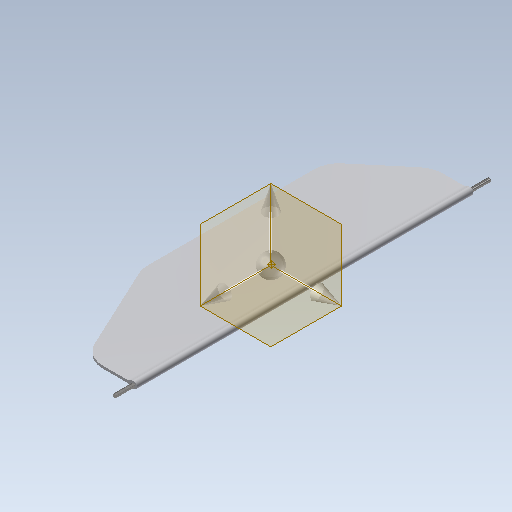
# Autodesk Inventor part: tail2
Saved by Autodesk Inventor 2020 (Build 240168000, 168)
## iProperties
Created: 2016-11-20
Part Number: tail2
Material: Generic
Document SubType Name: Modeling
Designer: jous
Density: 1 g/cm^3
Appearance: Default
Mass: 312.78 g
Surface Area: 1473.46 cm^2
Volume: 312.78 cm^3
sail_heightx: 1000.000 mm
tail_offsetx: 100.000 mm
Author: jous
Autodesk Inventor part; units mm, degrees
ref_plane "YZ Plane" through (0, 0, 0) normal (1, 0, 0) x (0, 1, 0)
ref_plane "XZ Plane" through (0, 0, 0) normal (0, 1, 0) x (-1, 0, 0)
ref_plane "XY Plane" through (0, 0, 0) normal (0, 0, 1) x (1, 0, 0)
sketch "Sketch1" plane through (0, 0, 0) normal (0, 0, 1) x (1, 0, 0)
  circle A0 centre (0, 0) radius 5.5
  circle A1 centre (0, 0) radius 3
  dimension "d0" = 11
  dimension "d1" = 6
  constraints: 2 centre point, 2 coincident
  measures "d0" diameter of A0
  measures "d1" diameter of A1
extrude "tube" add sketch "Sketch1" along normal blind 530
sketch "Sketch2" plane through (0, 0, 0) normal (0, 1, 0) x (-1, 0, 0)
  line L0 (0, 0) -> (150, 0)
  line L1 (150, 0) -> (150, 530)
  line L2 (150, 530) -> (0, 530)
  line L3 (0, 530) -> (0, 0)
  line L4 (75, 0) -> (165.4178, 0) construction
  line L5 (74, 530) -> (150, 367.0175)
  line L6 (74, 530) -> (253.8313, 530) construction
  line L7 (150, 77.1972) -> (58, 0)
  point P0 (150, 333)
  dimension "d4" = 150
  dimension "d5" = 530
  dimension "d9" = 65
  dimension "d16" = 74
  dimension "d17" = 58
  dimension "d18" = 40
  constraints: 16 end point, 5 point on line, 3 horizontal, 2 midpoint, 2 parallel, 1 equal length, 1 perpendicular
  measures "d4" distance of L2.end L1.end
  measures "d5" distance of L0.end L1.end
  measures "d9" angle of L5 L6
  measures "d16" distance of L2.end L5.start
  measures "d17" distance from line of L3 L7.end
  measures "d18" angle of L0 L7
extrude "tail" add sketch "Sketch2" along normal mid plane 4 contours L3 L2 L5 L1 L7 L0
fillet "Fillet1" radius 40 4 edges at (-74, 0, 530) (-150, 0, 367.0175) (-150, 0, 77.1972) (-58, 0, 0)
fillet "Fillet2" radius 20 2 edges at (-5.1235, -2, 265) (-5.1235, 2, 265)
extrude "shaft" add sketch "Sketch1" along normal blind 560 and the other way blind 30 contours A1
equation "\"d2\" = tail_height"
equation "\"d5\" = tail_height"
equation "\"tail_height\" = 530"
body "Solid1"
